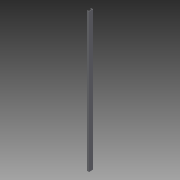
# Autodesk Inventor part: cChannel2x1-01
Saved by Autodesk Inventor 2013 (Build 170138000, 138)
## iProperties
Created: 2012-11-02
Part Number: cChannel2x1-01
Material: Generic
Document SubType Name: Modeling
Designer: istvan.burbank
Density: 1 g/cm^3
Author: istvan.burbank
Autodesk Inventor part; units mm, degrees
ref_plane "YZ Plane" through (0, 0, 0) normal (1, 0, 0) x (0, 1, 0)
ref_plane "XZ Plane" through (0, 0, 0) normal (0, 1, 0) x (-1, 0, 0)
ref_plane "XY Plane" through (0, 0, 0) normal (0, 0, 1) x (1, 0, 0)
sketch "Sketch1" plane through (0, 0, 0) normal (0, 1, 0) x (-1, 0, 0)
  line L0 (0, 0) -> (25.4, 0)
  line L1 (25.4, 50.8) -> (0, 50.8)
  line L2 (0, 50.8) -> (0, 0)
  line L3 (3.175, 3.175) -> (25.4, 3.175)
  line L4 (25.4, 47.625) -> (3.175, 47.625)
  line L5 (3.175, 47.625) -> (3.175, 3.175)
  line L6 (25.4, 0) -> (25.4, 3.175)
  line L7 (25.4, 47.625) -> (25.4, 50.8)
  dimension "d0" = 25.4
  dimension "d1" = 50.8
  dimension "d2" = 3.175
  dimension "d3" = 3.175
  constraints: 16 end point, 4 parallel, 2 perpendicular, 1 collinear, 1 horizontal, 1 other
  measures "d0" distance of L1.end L1.start
  measures "d1" distance of L1.start L0.end
  measures "d2" distance between parallel lines of L2 L5
  measures "d3" distance between parallel lines of L0 L3
extrude "Extrusion1" add sketch "Sketch1" along normal blind 1828.8
equation "\"d3\" = d2"
body "Solid1"
